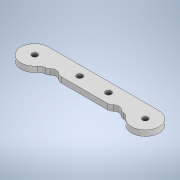
# Autodesk Inventor part: prig to kauri conversion plate
Saved by Autodesk Inventor 2020 (Build 240168000, 168)
## iProperties
Created: 2022-05-24
Part Number: prig to kauri conversion plate
Material: Generic
Document SubType Name: Modeling
Designer: Steven
Density: 1 g/cm^3
Appearance: Default
Author: Steven
Autodesk Inventor part; units mm, degrees
ref_plane "YZ Plane" through (0, 0, 0) normal (1, 0, 0) x (0, 1, 0)
ref_plane "XZ Plane" through (0, 0, 0) normal (0, 1, 0) x (-1, 0, 0)
ref_plane "XY Plane" through (0, 0, 0) normal (0, 0, 1) x (1, 0, 0)
sketch "Sketch1" plane through (0, 0, 0) normal (0, 1, 0) x (-1, 0, 0)
  circle A0 centre (-16.9706, -0.5878) radius 1.5
  circle A1 centre (16.9706, -0.5878) radius 1.5
  circle A2 centre (30, -5.1319) radius 1.5
  circle A3 centre (-30, -5.1319) radius 1.5
  circle A4 centre (16.9706, -0.5878) radius 5 construction
  circle A5 centre (-16.9706, -0.5878) radius 5 construction
  arc A6 (-31.1155, 2.2846) -> (-30, -12.6319) centre (-30, -5.1319) ccw
  arc A7 (30, -12.6319) -> (31.1155, 2.2846) centre (30, -5.1319) ccw
  line L0 (30, -12.6319) -> (-30, -12.6319)
  line L1 (-16.9706, 4.4122) -> (16.9706, 4.4122)
  line L2 (-16.9706, 4.4122) -> (-31.1155, 2.2846)
  line L3 (16.9706, 4.4122) -> (31.1155, 2.2846)
  arc A8 (31.1155, 2.2846) -> (23.1456, -2.0878) centre (30, -5.1319) ccw
  arc A9 (-30, -12.6319) -> (-23.1456, -2.0878) centre (-30, -5.1319) ccw construction
  line L4 (0, 4.2106) -> (0, -4.2106) construction
  line L5 (0, -4.2106) -> (3.1574, -4.2106) construction
  line L6 (0, -4.2106) -> (0, -12.6319) construction
  circle A10 centre (0, 0) radius 1.55
  line L7 (0, -8.4213) -> (15.6117, -8.4213) construction
  line L8 (0, -8.4213) -> (-15.6117, -8.4213) construction
  circle A11 centre (7.8058, -8.4213) radius 1.55 construction
  circle A12 centre (-7.8058, -8.4213) radius 1.55 construction
  line L9 (16.9706, -2.0878) -> (-16.9706, -2.0878)
  line L10 (16.9706, -2.0878) -> (23.1456, -2.0878)
  line L11 (-16.9706, -2.0878) -> (-23.1456, -2.0878)
  arc A13 (-23.1456, -2.0878) -> (-31.1155, 2.2846) centre (-30, -5.1319) ccw
  arc A14 (23.1456, -2.0878) -> (30, -12.6319) centre (30, -5.1319) ccw construction
  line L12 (7.8058, -12.6319) -> (7.8058, -2.0878) construction
  line L13 (-7.8058, -12.6319) -> (-7.8058, -2.0878) construction
  line L14 (3.5375, -12.6319) -> (3.5375, -2.0878) construction
  line L15 (3.5375, -7.3599) -> (10.9646, -7.3599) construction
  line L16 (3.5375, -7.3599) -> (-12.9158, -7.3599) construction
  circle A15 centre (7.8058, -7.3599) radius 1.55
  circle A16 centre (-7.8058, -7.3599) radius 1.55
  circle A17 centre (-16.9706, -0.5878) radius 3.25
  circle A18 centre (16.9706, -0.5878) radius 3.25
  circle A19 centre (16.9706, -0.5878) radius 2.75 construction
  line L17 (15.3828, -3.3378) -> (13.7951, -0.5878) construction
  line L18 (13.7951, -0.5878) -> (15.3828, 2.1622) construction
  line L19 (15.3828, 2.1622) -> (18.5583, 2.1622) construction
  line L20 (18.5583, 2.1622) -> (20.146, -0.5878) construction
  line L21 (20.146, -0.5878) -> (18.5583, -3.3378) construction
  line L22 (18.5583, -3.3378) -> (15.3828, -3.3378) construction
  point P0 (0, 0)
  point P1 (19.8537, -2.0878)
  point P2 (14.0874, -2.0878)
  point P3 (-14.0874, -2.0878)
  point P4 (-19.8537, -2.0878)
  point P5 (16.9706, -3.3378)
  dimension "d0" = 10
  dimension "d1" = 10
  dimension "d20" = 5.5
  dimension "d2" = 15
  dimension "d3" = 15
  dimension "d4" = 3.1
  dimension "d5" = 3.1
  dimension "d6" = 3.1
  dimension "d13" = 10.5442
  dimension "d14" = 3.1
  dimension "d15" = 3.1
  dimension "d16" = 6.5
  dimension "d17" = 6.5
  constraints: 46 end point, 15 centre point, 12 point on circle, 11 point on line, 9 midpoint, 8 coincident, 7 horizontal, 5 vertical alignment, 3 perpendicular, 3 tangent, 23 other
  measures "d2" diameter of A6
  measures "d3" diameter of A7
  measures "d4" diameter of A10
  measures "d5" diameter of A11
  measures "d6" diameter of A12
  measures "d13" distance of L14.start L14.end
  measures "d14" diameter of A15
  measures "d15" diameter of A16
  measures "d16" diameter of A17
  measures "d17" diameter of A18
extrude "Extrusion1" add sketch "Sketch1" along normal blind 3 contours L9 A18 L10 A8 A7 L0 A6 A13 L11 A17
fillet "Fillet2" radius 3 4 edges at (-19.8537, 1.5, -2.0878) (-14.0874, 1.5, -2.0878) (14.0874, 1.5, -2.0878) (19.8537, 1.5, -2.0878)
fillet "Fillet3" radius 4 2 edges at (-23.1456, 1.5, -2.0878) (23.1456, 1.5, -2.0878)
body "Solid1"
